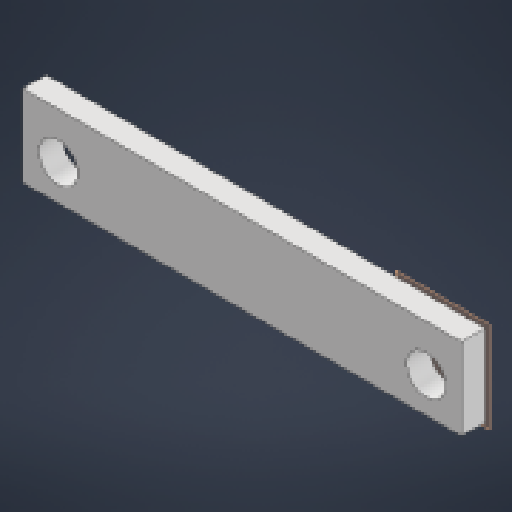
# Autodesk Inventor part: clip
Saved by Autodesk Inventor 2024.3 (Build 283343000, 343)
## iProperties
Created: 2025-08-15
Part Number: clip
Material: Generic
Document SubType Name: Modeling
Designer: giuseppe
Density: 1 g/cm^3
Appearance: Default
Author: giuseppe
Autodesk Inventor part; units mm, degrees
ref_plane "YZ Plane" through (0, 0, 0) normal (1, 0, 0) x (0, 1, 0)
ref_plane "XZ Plane" through (0, 0, 0) normal (0, 1, 0) x (-1, 0, 0)
ref_plane "XY Plane" through (0, 0, 0) normal (0, 0, 1) x (1, 0, 0)
ref_plane "Work Plane1" through (0, 0, 0) normal (0, 0, 1) x (1, 0, 0)
sketch "Sketch1" plane through (0, 0, 0) normal (0, 0, 1) x (1, 0, 0)
  circle A0 centre (-15.55, 1) radius 1.95 construction
  line L0 (-12.55, -11.9) -> (-12.55, -2) construction
  line L1 (-8.25, -11.9) -> (-12.55, -11.9) construction
  line L2 (-8.25, -10.7) -> (-8.25, -11.9) construction
  line L3 (-11.35, -10.7) -> (-8.25, -10.7) construction
  line L4 (-11.35, 4.9) -> (-11.35, -10.7) construction
  line L5 (-16.05, 4.9) -> (-11.35, 4.9) construction
  line L6 (-16.05, 3.8) -> (-16.05, 4.9) construction
  line L7 (-16.05, 3.8) -> (-18.55, 3.8) construction
  line L8 (-18.55, 3.8) -> (-18.55, -2) construction
  line L9 (-18.55, -2) -> (-12.55, -2) construction
  circle A1 centre (15.55, 1) radius 1.95 construction
  line L10 (11.35, -2) -> (11.35, 5) construction
  line L11 (18.55, -2) -> (11.35, -2) construction
  line L12 (18.55, 3.8) -> (18.55, -2) construction
  line L13 (16.05, 3.8) -> (18.55, 3.8) construction
  line L14 (16.05, 5) -> (16.05, 3.8) construction
  line L15 (11.35, 5) -> (16.05, 5) construction
  line L16 (-18.55, -2) -> (18.55, -2)
  line L17 (18.55, -2) -> (18.55, 4.9)
  line L18 (18.55, 4.9) -> (-18.55, 4.9)
  line L19 (-18.55, 4.9) -> (-18.55, -2)
  circle A2 centre (-15.55, 1) radius 1.65
  circle A3 centre (15.55, 1) radius 1.65
  point P0 (0, 0)
  dimension "d0" = 3.3
  constraints: 8 end point, 2 centre point, 2 coincident, 2 collinear, 2 parallel, 1 equal radius, 1 horizontal, 1 perpendicular
  measures "d0" diameter of A2
extrude "Extrusion1" add sketch "Sketch1" along normal blind 2
body "Solid1"
